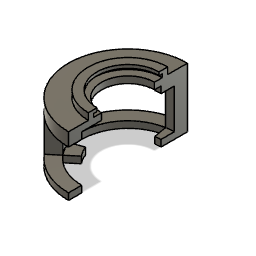
lamp holder v2 v3 (Autodesk Fusion 360 design; units mm, degrees)
Autodesk Fusion 360 part; units mm, degrees
sketch "Skizze1" plane through (0, 0, 0) normal (0, 1, 0) x (1, 0, 0)
  circle A0 centre (0, 0) radius 45
  circle A1 centre (0, 0) radius 35
  circle A2 centre (0, 0) radius 30
  arc A3 (-38.8822, -22.6534) -> (-28.7894, -34.5857) centre (0, 0) ccw
  arc A4 (39.0595, -22.3463) -> (44.3468, -7.6395) centre (0, 0) ccw
  arc A5 (7.8142, 44.3163) -> (-7.8142, 44.3163) centre (0, 0) ccw
  line L0 (0, 0) -> (7.8142, 44.3163)
  line L1 (0, 0) -> (-7.8142, 44.3163)
  line L2 (0, 45) -> (0, 0)
  circle A6 centre (0, 0) radius 25
  line L3 (0, 0) -> (-34.472, -28.9254)
  line L4 (0, 0) -> (-42.2862, -15.3909)
  line L5 (0, 0) -> (42.2862, -15.3909)
  line L6 (0, 0) -> (34.472, -28.9254)
  dimension "d1" = 90
  dimension "d2" = 70
  dimension "d3" = 60
  dimension "d8" = 20
  dimension "d9" = 50
  dimension "d11" = 360
  constraint coincident A0.centre A1.centre
  constraint concentric A0 A2
  constraint coincident A0 A5.end
  constraint coincident A5 L2.start
  constraint vertical L2
  constraint symmetric L0 L1 L2
  constraint concentric A3 A6
  measures "d1" diameter of A0
  measures "d2" diameter of A1
  measures "d3" diameter of A2
  measures "d8" angle of L0 L1
  measures "d9" diameter of A6
extrude "Extrusion1" add sketch "Skizze1" along normal blind 40 contours A0 A1 A4 L0 L5 | A0 A1 A5 L0 L2 | A0 A1 A5 L1 L2 | A1 A2 L0 L2 | A0 A1 A4 L5 L6 | A0 A1 L1 L4 | A1 A2 L1 L2 | A2 L0 L2 A6 | A1 A2 L5 L6 | A0 A1 A3 L3 L4 | A2 L1 L2 A6 | A0 A1 A3 L3 L6 | A2 A6 L5 L6 | A1 A2 L3 L4 | A2 A6 L3 L4 makes body 1
ref_plane "Arbeitsebene1" through (0, 5, 0) normal (0, 1, 0) x (0, 0, 1)
sketch "Skizze2" plane through (0, 5, 0) normal (0, 1, 0) x (1, 0, 0)
  circle A0 centre (0, 0) radius 35
  circle A1 centre (0, 0) radius 25
  line L0 (0, 45) -> (0, 0)
  line L1 (0, 0) -> (34.472, -28.9254)
  circle A2 centre (0, 0) radius 30
  arc A3 (39.0595, -22.3463) -> (44.3468, -7.6395) centre (0, 0) ccw
  arc A4 (-38.8822, -22.6534) -> (-28.7894, -34.5857) centre (0, 0) ccw
  circle A5 centre (0, 0) radius 35
  line L2 (0, 0) -> (-42.2862, -15.3909)
  arc A6 (7.8142, 44.3163) -> (-7.8142, 44.3163) centre (0, 0) ccw
  line L3 (0, 0) -> (7.8142, 44.3163)
  line L4 (0, 0) -> (-7.8142, 44.3163)
  line L5 (0, 0) -> (42.2862, -15.3909)
  line L6 (0, 0) -> (-34.472, -28.9254)
  circle A7 centre (0, 0) radius 45
  dimension "d15" = 70
  dimension "d19" = 360
  dimension "d20" = 90
  dimension "d21" = 70
  dimension "d22" = 60
  dimension "d23" = 20
  dimension "d24" = 50
  constraint coincident A0.centre A1.centre
  constraint concentric A2 A7
  constraint coincident A6.end A7
  constraint coincident L0.start A6
  constraint vertical L0
  constraint symmetric L0 L3 L4
  constraint concentric A1 A4
  measures "d15" diameter of A0
  measures "d20" diameter of A7
  measures "d21" diameter of A5
  measures "d22" diameter of A2
  measures "d23" angle of L3 L4
  measures "d24" diameter of A1
extrude "Extrusion2" cut sketch "Skizze2" along normal blind 30 contours A0 A3 A5 L3 L5 A7 | A0 L0 A2 A5 L3 | A0 L1 A2 A5 L5 | A0 L0 A2 A5 L4 | A1 L0 A2 L3 | A0 L1 A4 A5 L6 A7 | A1 L1 A2 L5 | A0 A5 L2 L4 A7 | A1 L0 A2 L4 | A0 A2 A5 L2 L6 | A1 A2 L2 L6 bodies 1
ref_plane "Arbeitsebene2" through (0, 40, 0) normal (0, 1, 0) x (0, 0, 1)
sketch "Skizze3" plane through (0, 40, 0) normal (0, 1, 0) x (1, 0, 0)
  circle A0 centre (0, 0) radius 45
  circle A1 centre (0, 0) radius 20
  dimension "d30" = 40
  dimension "d31" = 90
  constraint coincident A0.centre A1.centre
  measures "d30" diameter of A1
  measures "d31" diameter of A0
extrude "Extrusion4" add sketch "Skizze3" along normal blind 5 bodies 1
ref_plane "Arbeitsebene3" through (0, 45, 0) normal (0, 1, 0) x (0, 0, 1)
sketch "Skizze5" plane through (0, 45, 0) normal (0, 1, 0) x (1, 0, 0)
  circle A0 centre (0, 0) radius 23.5
  circle A1 centre (0, 0) radius 26
  circle A2 centre (0, 0) radius 30
  dimension "d36" = 47
  dimension "d37" = 52
  dimension "d44" = 60
  constraint coincident A0.centre A1.centre
  constraint concentric A0 A1
  measures "d36" diameter of A0
  measures "d37" diameter of A1
  measures "d44" diameter of A2
extrude "Extrusion7" add sketch "Skizze5" along normal blind 5 contours A0 | A1 | A2 bodies 1
ref_plane "Arbeitsebene4" through (0, 50, 0) normal (0, 1, 0) x (0, 0, 1)
sketch "Skizze6" plane through (0, 50, 0) normal (0, 1, 0) x (1, 0, 0)
  circle A0 centre (0, 0) radius 23.5
  dimension "d39" = 47
  constraint coincident A0.centre origin
  measures "d39" diameter of A0
extrude "Extrusion5" cut sketch "Skizze6" against normal blind 4 bodies 1
extrude "Extrusion6" cut sketch "Skizze5" along normal blind 2.5 contours A0 | A1 bodies 1
split "Teilen1" by plane through (0, 0, 0) normal (1, 0, 0) bodies 1 makes body 2 at (39.8473, 45, 2.1347)
